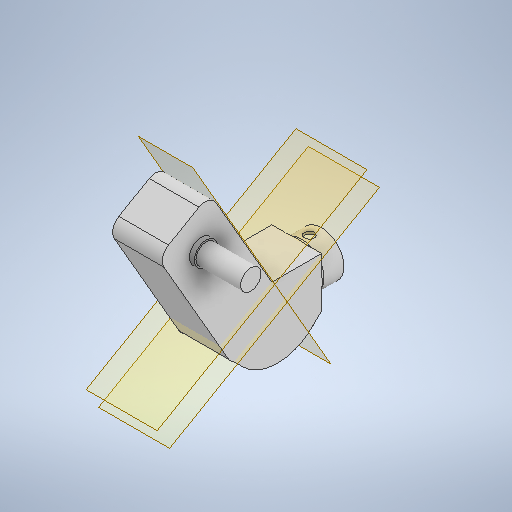
# Autodesk Inventor part: bielle roue milieu autre côté
Saved by Autodesk Inventor 2026.2 (Build 302298010, 298A)
## iProperties
Created: 2026-03-19
Part Number: bielle roue milieu autre côté
Material: Générique
Document SubType Name: Modeling
Designer: Genon
Density: 1 g/cm^3
Appearance: Par défaut
Author: Genon
Autodesk Inventor part; units mm, degrees
ref_plane "YZ Plane" through (0, 0, 0) normal (1, 0, 0) x (0, 1, 0)
ref_plane "XZ Plane" through (0, 0, 0) normal (0, 1, 0) x (-1, 0, 0)
sketch "Esquisse1" plane through (0, 0, 0) normal (0, 0, 1) x (1, 0, 0)
  circle A0 centre (0, 0) radius 8
  circle A1 centre (0, 0) radius 9
  dimension "d0" = 16
  dimension "d1" = 18
  constraints: 2 centre point, 2 coincident
  measures "d0" diameter of A0
  measures "d1" diameter of A1
extrude "Extrusion1" add sketch "Esquisse1" along normal blind 10
sketch "Esquisse2" plane through (0, 0, 0) normal (1, 0, 0) x (0, 1, 0)
  line L0 (9, 10) -> (-9, 10) projected
  line L1 (0, 10) -> (0, 25)
  line L2 (9, 10) -> (-9, 10)
  line L3 (0, 10) -> (10, 10)
  line L4 (10, 10) -> (10, 30)
  line L5 (10, 30) -> (-10, 30)
  line L6 (-10, 30) -> (-10, 10)
  line L7 (-10, 10) -> (0, 10)
  point P0 (0, 0)
  dimension "d26" = 10
  dimension "d27" = 20
  dimension "d28" = 20
  dimension "d29" = 90
  constraints: 14 end point, 3 perpendicular, 2 point on line, 1 collinear, 1 midpoint, 1 vertical
  measures "d26" distance of L1.start L3.end
  measures "d27" distance of L3.end L4.end
  measures "d28" distance of L4.end L5.end
  measures "d29" angle of L5 L4
extrude "Extrusion2" add sketch "Esquisse2" along normal mid plane 20
fillet "Congé1" radius 2 1 edges at (-9, 0, 10)
sketch "Esquisse4" plane through (0, 0, 0) normal (0, 1, 0) x (-1, 0, 0)
  line L0 (9, 0) -> (-9, 0) projected
  line L1 (9, 0) -> (0, 0)
  line L2 (0, 0) -> (0, 5)
  line L3 (0, 0) -> (5, 0) construction
  dimension "d14" = 9
  dimension "d15" = 5
  dimension "d16" = 90
  constraints: 6 end point, 2 perpendicular, 1 coincident, 1 collinear, 1 horizontal
  measures "d14" distance of L0.start L1.end
  measures "d15" distance of L1.end L2.end
  measures "d16" angle of L3 L2
hole "Perçage1" at (0, 0, 5) direction (0, -1, 0) diameter 4 end through all both
ref_plane "Plan de construction2" through (0, -8.75, 15.1554) normal (0, -0.5, 0.8660254) x (1, 0, 0)
ref_plane "Plan de construction1" through (0, 0, 0) normal (0, -0.5, 0.8660254) x (1, 0, 0)
ref_plane "Plan de construction4" through (0, -10, 10) normal (0, -0.7071068, 0.7071068) x (1, 0, 0)
ref_plane "Plan de construction3" through (0, 0, 0) normal (0, -0.7071068, 0.7071068) x (1, 0, 0)
sketch "Esquisse6" plane through (0, -10, 10) normal (0, -0.7071068, 0.7071068) x (1, 0, 0)
  line L0 (-10, 28.2843) -> (-10, 14.1421) projected
  line L1 (10, 14.1421) -> (10, 0) projected
  line L2 (-10, 28.2843) -> (10, 28.2843)
  line L3 (10, 28.2843) -> (10, 0)
  line L4 (10, 0) -> (-10, 0)
  line L5 (-10, 0) -> (-10, 28.2843)
  line L6 (-10, 28.2843) -> (10, 28.2843) projected
  line L7 (10, 14.1421) -> (10, 28.2843) projected
  line L8 (4.5826, 14.1421) -> (10, 14.1421) projected
  line L9 (-10, 14.1421) -> (-4.5826, 14.1421) projected
  line L10 (-10, 28.2843) -> (-10, 14.1421) projected
  point P0 (0, 0)
  constraints: 8 end point, 2 parallel, 1 horizontal, 1 horizontal alignment, 1 perpendicular
extrude "Extrusion4" add sketch "Esquisse6" along normal blind 25
fillet "Congé4" radius 20 1 edges at (0, -27.6777, 27.6777)
ref_plane "Plan de construction5" through (0, 10, 30) normal (0, 0.8660254, 0.5) x (1, 0, 0)
ref_plane "Plan de construction7" through (0, 10, 30) normal (0, -0.5, 0.8660254) x (1, 0, 0)
ref_plane "Plan de construction6" through (0, 1.3397, 25) normal (0, 0.8660254, 0.5) x (1, 0, 0)
sketch "Esquisse18" plane through (0, 1.3397, 25) normal (0, 0.8660254, 0.5) x (1, 0, 0)
  line L0 (10, -0.0001) -> (-10, -0.0001) projected
  line L1 (-10, -0.0001) -> (-10, -24.1482) projected
  line L2 (10, -24.1482) -> (-10, -24.1482) projected
  line L3 (10, -0.0001) -> (10, -24.1482) projected
  line L4 (10, -0.0001) -> (-10, -0.0001) projected
  line L5 (-10, -0.0001) -> (-10, -24.1482) projected
  line L6 (10, -24.1482) -> (-10, -24.1482) projected
  line L7 (10, -0.0001) -> (10, -24.1482) projected
  point P0 (0, 20.9808)
extrude "Extrusion14" add sketch "Esquisse18" along normal blind 60
fillet "Congé6" radius 5 1 edges at (0, -10.7344, 45.913)
sketch "Esquisse19" plane through (10, 0, 0) normal (1, 0, 0) x (0, 0, -1)
  line L0 (-30, 10) -> (-55.0001, 53.3012) projected
  line L1 (-55.0001, 53.3012) -> (-65.4564, 47.2642)
  line L2 (-47.3761, -8.2002) -> (-75.913, 41.2272) projected
  line L3 (-65.4564, 47.2642) -> (-58.4714, 35.1659)
  circle A0 centre (-58.4714, 35.1659) radius 4.1
  point P0 (0, 0)
  dimension "d76" = 12.074
  dimension "d77" = 13.97
  dimension "d78" = 8.2
  constraints: 4 end point, 2 perpendicular, 1 centre point, 1 coincident
  measures "d76" distance of L0.end L1.end
  measures "d77" distance of L1.end L3.end
  measures "d78" diameter of A0
extrude "Extrusion15" add sketch "Esquisse19" along normal blind 20
sketch "Esquisse20" plane through (10, 0, 0) normal (1, 0, 0) x (0, 0, -1)
  circle A0 centre (-58.4714, 35.1659) radius 4.1 projected
  circle A1 centre (-58.4714, 35.1659) radius 4.75
  point P0 (0, 0)
  dimension "d81" = 9.5
  constraints: 1 centre point, 1 coincident
  measures "d81" diameter of A1
extrude "Extrusion16" add sketch "Esquisse20" along normal blind 2
fillet "Congé7" radius 5 2 edges at (0, 53.3012, 55.0001) (0, 41.2272, 75.913)
